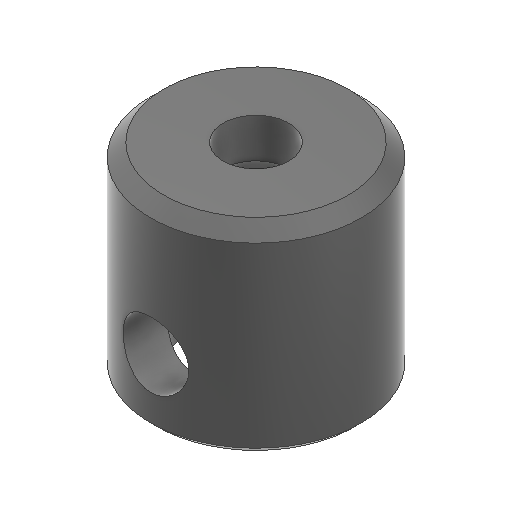
# Autodesk Inventor part: acople_iman
Saved by Autodesk Inventor 2025 (Build 290162000, 162)
## iProperties
Created: 2026-02-07
Part Number: acople_iman
Material: Genérico
Document SubType Name: Modeling
Designer: HP
Density: 1 g/cm^3
Appearance: Valor por defecto
Author: HP
Autodesk Inventor part; units mm, degrees
ref_plane "YZ Plane" through (0, 0, 0) normal (1, 0, 0) x (0, 1, 0)
ref_plane "Plano de trabajo1" through (18.3204, 15.1618, 2.5684) normal (0, 1, 0) x (-1, 0, 0)
sketch "Boceto1" plane through (18.3204, 15.1618, 2.5684) normal (0, 1, 0) x (-1, 0, 0)
  circle A0 centre (0, 0) radius 5 projected
  circle A1 centre (0, 0) radius 8
  point P0 (18.3204, -2.5684)
  dimension "d0" = 3
  constraints: 1 centre point
  measures "d0" radial gap between concentric circles of A0 A1
extrude "Extrusión1" add sketch "Boceto1" along normal blind 5 and the other way blind 5
sketch "Boceto2" plane through (18.3204, 20.1618, 2.5684) normal (0, 1, 0) x (1, 0, 0)
  circle A0 centre (0, 0) radius 8 projected
  point P0 (-18.3204, 2.5684)
extrude "Extrusión2" add sketch "Boceto2" along normal blind 5
sketch "Boceto3" plane through (18.3204, 25.1618, 2.5684) normal (0, 1, 0) x (1, 0, 0)
  circle A0 centre (0, 0) radius 2.5
  point P0 (-18.3204, 2.5684)
  dimension "d7" = 5
  constraints: 1 centre point
  measures "d7" diameter of A0
extrude "Extrusión3" cut sketch "Boceto3" against normal blind 3
ref_plane "Plano de trabajo2" through (0, 0, 11) normal (0, 0, 1) x (1, 0, 0)
sketch "Boceto4" plane through (0, 0, 11) normal (0, 0, 1) x (1, 0, 0)
  line L0 (26.3204, 25.1618) -> (10.3204, 25.1618) projected
  line L1 (10.3204, 10.1618) -> (26.3204, 10.1618) projected
  circle A0 centre (18.3204, 15.1618) radius 2.5
  point P0 (0, 0)
  dimension "d11" = 5
  dimension "d12" = 5
  constraints: 1 centre point
  measures "d11" diameter of A0
  measures "d12" distance from line of A0.centre L1
extrude "Extrusión4" cut sketch "Boceto4" against normal blind 6
chamfer "Chaflán1" distance 0.5 angle 45 1 edges at (26.3204, 10.1618, 2.5684)
chamfer "Chaflán2" distance 1 angle 45 1 edges at (10.3204, 25.1618, 2.5684)
